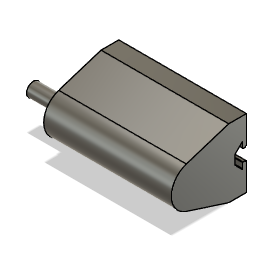
Washer Support v6 (Autodesk Fusion 360 design; units mm, degrees)
Autodesk Fusion 360 part; units mm, degrees
sketch "Sketch1" plane through (0, 0, 0) normal (0, 0, 1) x (1, 0, 0)
  line L0 (0, 0) -> (60, 0)
  line L1 (60, 0) -> (60, 38)
  line L2 (60, 38) -> (0, 38)
  line L3 (0, 38) -> (0, 0)
  point P0 (0, 19)
  dimension "d1" = 38
  dimension "d10" = 60
  constraint horizontal L0
  constraint vertical L1
  constraint horizontal L2
  constraint vertical L3
  constraint coincident L0.start L3.end
  constraint midpoint L3 P0
  measures "d1" distance of L0.start L2.end
  measures "d10" distance of L1.end L2.end
extrude "Extrude1" add sketch "Sketch1" along normal blind 57 makes body 1
sketch "Sketch2" plane through (0, 0, 0) normal (-1, 0, 0) x (0, 0, 1)
  line L0 (0, 38) -> (0, 0)
  line L1 (0, 0) -> (57, 0)
  line L2 (57, 0) -> (57, 38)
  line L3 (57, 38) -> (0, 38)
  line L4 (0, 38) -> (57, 0) construction
  circle A0 centre (28.5, 19) radius 3.85
  line L5 (0, 10) -> (0, 38)
  line L6 (57, 38) -> (0, 38)
  line L7 (57, 38) -> (57, 10)
  line L8 (28.5, 15.15) -> (57, 15.15) construction
  line L9 (28.5, 22.85) -> (57, 22.85) construction
  line L10 (9.8511, 38) -> (57, 22.85)
  line L11 (9.8511, 0) -> (57, 15.15)
  line L12 (57, 22.85) -> (33.4265, 30.4247)
  line L13 (57, 15.15) -> (33.4265, 7.5753)
  arc A1 (33.4265, 7.5753) -> (33.4265, 30.4247) centre (29.7555, 19) ccw
  line L14 (0, 38) -> (57, 38)
  line L15 (57, 38) -> (57, 0)
  line L16 (57, 0) -> (0, 0)
  line L17 (0, 0) -> (0, 38)
  point P0 (9.8511, 38)
  point P1 (9.8511, 0)
  dimension "d4" = 7.7
  dimension "d11" = 12
  constraint coincident L0.start L3.end
  constraint coincident L1.end L2.start
  constraint midpoint L4 A0.centre
  constraint coincident L0 L5.start
  constraint coincident L2 L7.end
  constraint coincident L2.end L3.start
  constraint coincident L6 P0
  constraint coincident L1 P1
  constraint coincident A0 L8.start
  constraint coincident L7 L8.end
  constraint coincident A0 L9.start
  constraint coincident L7 L9.end
  constraint perpendicular L7 L9
  constraint perpendicular L7 L8
  constraint tangent A0 L9
  constraint tangent A0 L8
  constraint coincident P0 L10.start
  constraint coincident P1 L11.start
  constraint collinear L10 L12
  constraint collinear L11 L13
  constraint tangent L13 A1
  constraint tangent L12 A1
  constraint horizontal L14
  constraint vertical L15
  constraint horizontal L16
  constraint vertical L17
  measures "d4" diameter of A0
  measures "d11" radius of A1
extrude "Extrude2" add sketch "Sketch2" along normal blind 19 contours A0 bodies 1
extrude "Extrude4" cut sketch "Sketch2" against normal blind 93 contours L2 L3 L6 L7 L10 L12 L14 L15 | L2 L7 L10 L11 L12 L13 A1 L15 | L1 L2 L7 L11 L13 L15 L16 bodies 1
sketch "profile" plane through (0, 0, 0) normal (0, 1, 0) x (1, 0, 0) in component "20 mm x 20 mm T-Slot v1"
  circle A0 centre (0, 0) radius 2.5
  line L0 (0, -3.9) -> (-2.5, -3.9)
  line L1 (4, -4) -> (-4, 4) construction
  line L2 (-3.9092, -3.9092) -> (4, 4) construction
  line L3 (10, -10) -> (-10, -10) construction
  line L4 (-10, -10) -> (-10, 10) construction
  line L5 (-10, 10) -> (10, 10) construction
  line L6 (10, 10) -> (10, -10) construction
  line L7 (10, -10) -> (-10, 10) construction
  line L8 (-10, -10) -> (10, 10) construction
  line L9 (8, -8) -> (-8, -8) construction
  line L10 (-8, -8) -> (-8, 8) construction
  line L11 (-8, 8) -> (8, 8) construction
  line L12 (8, 8) -> (8, -8) construction
  line L13 (8, -8) -> (-8, 8) construction
  line L14 (-8, -8) -> (8, 8) construction
  line L15 (0, -8) -> (0, -10) construction
  line L16 (0, -9) -> (-3.1, -9) construction
  line L17 (-3.1, -8) -> (-3.1, -9.6)
  line L18 (-1.75, -10) -> (-1.75, -9.6) construction
  line L19 (0, -9.6) -> (-3.5, -9.6) construction
  line L20 (-3.1, -9.6) -> (-3.5, -9.6)
  line L21 (-3.5, -9.6) -> (-3.5, -10)
  line L22 (0, 0) -> (0, -8) construction
  line L23 (-3.5, -10) -> (-10, -10)
  line L24 (-3.9092, -3.9092) -> (-2.5, -3.9) construction
  line L25 (-8, -8) -> (-6.6, -8) construction
  line L26 (-8, -8) -> (-8, -7) construction
  line L27 (-2.5, -3.9) -> (-6.6, -8)
  line L28 (-6.6, -8) -> (-3.1, -8)
  line L29 (0, -2.5) -> (0, -3.9) construction
  line L30 (-3.9, 0) -> (-3.9, -2.5)
  line L31 (-3.9, -2.5) -> (-8, -6.6)
  line L32 (-8, -6.6) -> (-8, -3.1)
  line L33 (-8, -3.1) -> (-9.6, -3.1)
  line L34 (-9.6, -3.1) -> (-9.6, -3.5)
  line L35 (-9.6, -3.5) -> (-10, -3.5)
  line L36 (-10, -3.5) -> (-10, -10)
  line L37 (0, 0) -> (10, 0) construction
  line L38 (3.9, 0) -> (3.9, -2.5)
  line L39 (3.9, -2.5) -> (8, -6.6)
  line L40 (8, -6.6) -> (8, -3.1)
  line L41 (8, -3.1) -> (9.6, -3.1)
  line L42 (9.6, -3.1) -> (9.6, -3.5)
  line L43 (9.6, -3.5) -> (10, -3.5)
  line L44 (10, -3.5) -> (10, -10)
  line L45 (0, -3.9) -> (2.5, -3.9)
  line L46 (6.6, -8) -> (3.1, -8)
  line L47 (3.1, -8) -> (3.1, -9.6)
  line L48 (3.1, -9.6) -> (3.5, -9.6)
  line L49 (3.5, -9.6) -> (3.5, -10)
  line L50 (3.5, -10) -> (10, -10)
  line L51 (2.5, -3.9) -> (6.6, -8)
  line L52 (-3.9, 0) -> (-3.9, 2.5)
  line L53 (-3.9, 2.5) -> (-8, 6.6)
  line L54 (-8, 6.6) -> (-8, 3.1)
  line L55 (-8, 3.1) -> (-9.6, 3.1)
  line L56 (-9.6, 3.1) -> (-9.6, 3.5)
  line L57 (-9.6, 3.5) -> (-10, 3.5)
  line L58 (-10, 3.5) -> (-10, 10)
  line L59 (0, 3.9) -> (-2.5, 3.9)
  line L60 (-6.6, 8) -> (-3.1, 8)
  line L61 (-3.1, 8) -> (-3.1, 9.6)
  line L62 (-3.1, 9.6) -> (-3.5, 9.6)
  line L63 (-3.5, 9.6) -> (-3.5, 10)
  line L64 (-3.5, 10) -> (-10, 10)
  line L65 (-2.5, 3.9) -> (-6.6, 8)
  line L66 (0, 3.9) -> (2.5, 3.9)
  line L67 (6.6, 8) -> (3.1, 8)
  line L68 (3.1, 8) -> (3.1, 9.6)
  line L69 (3.1, 9.6) -> (3.5, 9.6)
  line L70 (3.5, 9.6) -> (3.5, 10)
  line L71 (3.5, 10) -> (10, 10)
  line L72 (2.5, 3.9) -> (6.6, 8)
  line L73 (3.9, 0) -> (3.9, 2.5)
  line L74 (8, 6.6) -> (8, 3.1)
  line L75 (8, 3.1) -> (9.6, 3.1)
  line L76 (9.6, 3.1) -> (9.6, 3.5)
  line L77 (9.6, 3.5) -> (10, 3.5)
  line L78 (10, 3.5) -> (10, 10)
  line L79 (3.9, 2.5) -> (8, 6.6)
  dimension "d3_1" = 5
  dimension "d7" = 8
  dimension "d8" = 8
  dimension "d9" = 20
  dimension "d10_1" = 20
  dimension "d11_1" = 16
  dimension "d12_1" = 16
  dimension "d13_1" = 3.1
  dimension "d14" = 0.4
  dimension "d15" = 3.5
  dimension "d20" = 2.5
  dimension "d21" = 1.4
  constraint coincident A0.centre L22.start
  constraint horizontal L0
  constraint coincident L1 A0.centre
  constraint coincident L2 A0.centre
  constraint horizontal L3
  constraint perpendicular L3 L4
  constraint parallel L3 L5
  constraint parallel L4 L6
  constraint coincident L7 A0.centre
  constraint coincident L8 A0.centre
  constraint horizontal L9
  constraint perpendicular L9 L10
  constraint parallel L9 L11
  constraint parallel L10 L12
  constraint coincident L13 A0.centre
  constraint coincident L14 A0.centre
  constraint midpoint L9 L15.start
  constraint midpoint L3 L15.end
  constraint midpoint L15 L16.start
  constraint perpendicular L15 L16
  constraint coincident L9 L17.start
  constraint perpendicular L3 L17
  constraint coincident L16.end L17
  constraint vertical L18
  constraint coincident L3 L18.start
  constraint coincident L15 L19.start
  constraint perpendicular L15 L19
  constraint coincident L18.end L19
  constraint coincident L19 L17.end
  constraint coincident L3 L21.end
  constraint perpendicular L3 L21
  constraint midpoint L18.end L19
  constraint coincident L9 L25.end
  constraint coincident L10 L26.end
  constraint parallel L14 L27
  constraint coincident L22 L0.start
  constraint coincident L22 L29.start
  constraint coincident A0 L29.start
  constraint parallel L22 L29
  constraint coincident L0.start L29.end
  constraint symmetric L3.end L8 L4.start
  constraint symmetric L8 L17.start L32.end
  constraint symmetric L8 L19.end L34.end
  constraint symmetric L8 L17.end L33.end
  constraint symmetric L8 L21.end L35.end
  constraint symmetric L8 L0.end L30.end
  constraint symmetric L8 L25.end L31.end
  constraint symmetric L8 L0.start L30.start
  constraint midpoint L6 L37.end
  constraint symmetric L3.end L22 L3.start
  constraint symmetric L17.start L22 L46.end
  constraint symmetric L19.end L22 L48.end
  constraint symmetric L17.end L22 L47.end
  constraint symmetric L21.end L22 L49.end
  constraint symmetric L22 L0.end L45.end
  constraint symmetric L22 L25.end L46.start
  constraint symmetric L22 L0.start L29.end
  constraint symmetric L22 L30.start L38.start
  constraint symmetric L22 L30.end L38.end
  constraint symmetric L22 L31.end L39.end
  constraint symmetric L22 L32.end L40.end
  constraint symmetric L22 L33.end L41.end
  constraint symmetric L22 L34.end L42.end
  constraint symmetric L22 L35.end L43.end
  constraint symmetric L22 L3.end L3.start
  constraint symmetric L3.end L37 L4.end
  constraint symmetric L17.start L37 L60.end
  constraint symmetric L19.end L37 L62.end
  constraint symmetric L17.end L37 L61.end
  constraint symmetric L21.end L37 L63.end
  constraint symmetric L0.end L37 L59.end
  constraint symmetric L25.end L37 L60.start
  constraint symmetric L0.start L37 L59.start
  constraint symmetric L30.start L37 L52.start
  constraint symmetric L30.end L37 L52.end
  constraint symmetric L31.end L37 L53.end
  constraint symmetric L32.end L37 L54.end
  constraint symmetric L33.end L37 L55.end
  constraint symmetric L34.end L37 L56.end
  constraint symmetric L35.end L37 L57.end
  constraint symmetric L37 L38.start L73.start
  constraint symmetric L37 L38.end L73.end
  constraint symmetric L37 L39.end L74.start
  constraint symmetric L37 L40.end L74.end
  constraint symmetric L37 L41.end L75.end
  constraint symmetric L37 L42.end L76.end
  constraint symmetric L37 L43.end L77.end
  constraint symmetric L37 L3.start L5.end
  constraint symmetric L37 L0.start L59.start
  constraint symmetric L37 L45.end L66.end
  constraint symmetric L37 L46.start L67.start
  constraint symmetric L37 L46.end L67.end
  constraint symmetric L37 L47.end L68.end
  constraint symmetric L37 L48.end L69.end
  constraint symmetric L37 L49.end L70.end
  measures "d3_1" diameter of A0
  measures "d7" distance of L1.end L2.end
  measures "d8" distance of L1.start L2.end
  measures "d9" distance of L4.end L5.end
  measures "d10_1" distance of L3.end L4.end
  measures "d11_1" distance of L10.end L11.end
  measures "d12_1" distance of L9.end L10.end
  measures "d13_1" distance of L16.start L16.end
  measures "d14" distance of L18.start L18.end
  measures "d15" distance of L19.start L19.end
  measures "d20" distance of L0.end L0.start
  measures "d21" distance of L29.start L0.start
extrude "Extrude3" add sketch "profile" along normal blind 10 separate body makes body 2 in component "20 mm x 20 mm T-Slot v1"
fillet "Fillet1" radius 0.6 4 edges at (-10, 5, 10) (10, 5, 10) (10, 5, -10) (-10, 5, -10) on bodies 2 in component "20 mm x 20 mm T-Slot v1"
fillet "Fillet1" radius 0.2 8 edges at (3.1, 5, 8) (8, 5, 3.1) (8, 5, -3.1) (3.1, 5, -8) (-3.1, 5, 8) (-8, 5, 3.1) (-3.1, 5, -8) (-8, 5, -3.1) on bodies 2 in component "20 mm x 20 mm T-Slot v1"
fillet "Fillet1" radius 0.2 8 edges at (-8, 5, 6.6) (-6.6, 5, 8) (6.6, 5, 8) (8, 5, 6.6) (8, 5, -6.6) (6.6, 5, -8) (-6.6, 5, -8) (-8, 5, -6.6) on bodies 2 in component "20 mm x 20 mm T-Slot v1"
fillet "Fillet1" radius 0.4 8 edges at (-2.5, 5, 3.9) (2.5, 5, 3.9) (3.9, 5, 2.5) (3.9, 5, -2.5) (2.5, 5, -3.9) (-2.5, 5, -3.9) (-3.9, 5, -2.5) (-3.9, 5, 2.5) on bodies 2 in component "20 mm x 20 mm T-Slot v1"
scale "Scale1" factor 1.05 about (-2.3343, 10, 3.9) bodies 2 in component "20 mm x 20 mm T-Slot v1"
sketch "Sketch3" plane through (85, 0, 0) normal (1, 0, 0) x (0, 0, -1)
  arc A0 (-7.21, 27.4933) -> (-7, 27.2833) centre (-7, 27.4933) ccw
  line L0 (-7, 27.2833) -> (-4.042, 27.2833)
  arc A1 (-3.8935, 26.9248) -> (-4.042, 27.2833) centre (-4.042, 27.0733) ccw
  line L1 (-3.8935, 26.9248) -> (-7.717, 23.1013)
  arc A2 (-8.014, 22.9783) -> (-7.717, 23.1013) centre (-8.014, 23.3983) ccw
  line L2 (-8.014, 22.9783) -> (-12.916, 22.9783)
  arc A3 (-13.213, 23.1013) -> (-12.916, 22.9783) centre (-12.916, 23.3983) ccw
  line L3 (-13.213, 23.1013) -> (-17.0365, 26.9248)
  arc A4 (-16.888, 27.2833) -> (-17.0365, 26.9248) centre (-16.888, 27.0733) ccw
  line L4 (-16.888, 27.2833) -> (-13.93, 27.2833)
  arc A5 (-13.93, 27.2833) -> (-13.72, 27.4933) centre (-13.93, 27.4933) ccw
  line L5 (-13.72, 27.4933) -> (-13.72, 28.9633)
  line L6 (-13.72, 28.9633) -> (-14.14, 28.9633)
  line L7 (-14.14, 28.9633) -> (-14.14, 29.3833)
  line L8 (-14.14, 29.3833) -> (-20.335, 29.3833)
  arc A6 (-20.335, 29.3833) -> (-20.965, 28.7533) centre (-20.335, 28.7533) ccw
  line L9 (-20.965, 28.7533) -> (-20.965, 22.5583)
  line L10 (-20.965, 22.5583) -> (-20.545, 22.5583)
  line L11 (-20.545, 22.5583) -> (-20.545, 22.1383)
  line L12 (-20.545, 22.1383) -> (-19.075, 22.1383)
  arc A7 (-19.075, 22.1383) -> (-18.865, 22.3483) centre (-19.075, 22.3483) ccw
  line L13 (-18.865, 22.3483) -> (-18.865, 25.3063)
  arc A8 (-18.5065, 25.4548) -> (-18.865, 25.3063) centre (-18.655, 25.3063) ccw
  line L14 (-18.5065, 25.4548) -> (-14.683, 21.6313)
  arc A9 (-14.56, 21.3343) -> (-14.683, 21.6313) centre (-14.98, 21.3343) ccw
  line L15 (-14.56, 21.3343) -> (-14.56, 16.4323)
  arc A10 (-14.683, 16.1353) -> (-14.56, 16.4323) centre (-14.98, 16.4323) ccw
  line L16 (-14.683, 16.1353) -> (-18.5065, 12.3118)
  arc A11 (-18.865, 12.4603) -> (-18.5065, 12.3118) centre (-18.655, 12.4603) ccw
  line L17 (-18.865, 12.4603) -> (-18.865, 15.4183)
  arc A12 (-18.865, 15.4183) -> (-19.075, 15.6283) centre (-19.075, 15.4183) ccw
  line L18 (-19.075, 15.6283) -> (-20.545, 15.6283)
  line L19 (-20.545, 15.6283) -> (-20.545, 15.2083)
  line L20 (-20.545, 15.2083) -> (-20.965, 15.2083)
  line L21 (-20.965, 15.2083) -> (-20.965, 9.0133)
  arc A13 (-20.965, 9.0133) -> (-20.335, 8.3833) centre (-20.335, 9.0133) ccw
  line L22 (-20.335, 8.3833) -> (-14.14, 8.3833)
  line L23 (-14.14, 8.3833) -> (-14.14, 8.8033)
  line L24 (-14.14, 8.8033) -> (-13.72, 8.8033)
  line L25 (-13.72, 8.8033) -> (-13.72, 10.2733)
  arc A14 (-13.72, 10.2733) -> (-13.93, 10.4833) centre (-13.93, 10.2733) ccw
  line L26 (-13.93, 10.4833) -> (-16.888, 10.4833)
  arc A15 (-17.0365, 10.8418) -> (-16.888, 10.4833) centre (-16.888, 10.6933) ccw
  line L27 (-17.0365, 10.8418) -> (-13.213, 14.6653)
  arc A16 (-12.916, 14.7883) -> (-13.213, 14.6653) centre (-12.916, 14.3683) ccw
  line L28 (-12.916, 14.7883) -> (-8.014, 14.7883)
  arc A17 (-7.717, 14.6653) -> (-8.014, 14.7883) centre (-8.014, 14.3683) ccw
  line L29 (-7.717, 14.6653) -> (-3.8935, 10.8418)
  arc A18 (-4.042, 10.4833) -> (-3.8935, 10.8418) centre (-4.042, 10.6933) ccw
  line L30 (-4.042, 10.4833) -> (-7, 10.4833)
  arc A19 (-7, 10.4833) -> (-7.21, 10.2733) centre (-7, 10.2733) ccw
  line L31 (-7.21, 10.2733) -> (-7.21, 8.8033)
  line L32 (-7.21, 8.8033) -> (-6.79, 8.8033)
  line L33 (-6.79, 8.8033) -> (-6.79, 8.3833)
  line L34 (-6.79, 8.3833) -> (-0.595, 8.3833)
  arc A20 (-0.595, 8.3833) -> (0.035, 9.0133) centre (-0.595, 9.0133) ccw
  line L35 (0.035, 9.0133) -> (0.035, 15.2083)
  line L36 (0.035, 15.2083) -> (-0.385, 15.2083)
  line L37 (-0.385, 15.2083) -> (-0.385, 15.6283)
  line L38 (-0.385, 15.6283) -> (-1.855, 15.6283)
  arc A21 (-1.855, 15.6283) -> (-2.065, 15.4183) centre (-1.855, 15.4183) ccw
  line L39 (-2.065, 15.4183) -> (-2.065, 12.4603)
  arc A22 (-2.4235, 12.3118) -> (-2.065, 12.4603) centre (-2.275, 12.4603) ccw
  line L40 (-2.4235, 12.3118) -> (-6.247, 16.1353)
  arc A23 (-6.37, 16.4323) -> (-6.247, 16.1353) centre (-5.95, 16.4323) ccw
  line L41 (-6.37, 16.4323) -> (-6.37, 21.3343)
  arc A24 (-6.247, 21.6313) -> (-6.37, 21.3343) centre (-5.95, 21.3343) ccw
  line L42 (-6.247, 21.6313) -> (-2.4235, 25.4548)
  arc A25 (-2.065, 25.3063) -> (-2.4235, 25.4548) centre (-2.275, 25.3063) ccw
  line L43 (-2.065, 25.3063) -> (-2.065, 22.3483)
  arc A26 (-2.065, 22.3483) -> (-1.855, 22.1383) centre (-1.855, 22.3483) ccw
  line L44 (-1.855, 22.1383) -> (-0.385, 22.1383)
  line L45 (-0.385, 22.1383) -> (-0.385, 22.5583)
  line L46 (-0.385, 22.5583) -> (0.035, 22.5583)
  line L47 (0.035, 22.5583) -> (0.035, 28.7533)
  arc A27 (0.035, 28.7533) -> (-0.595, 29.3833) centre (-0.595, 28.7533) ccw
  line L48 (-0.595, 29.3833) -> (-6.79, 29.3833)
  line L49 (-6.79, 29.3833) -> (-6.79, 28.9633)
  line L50 (-6.79, 28.9633) -> (-7.21, 28.9633)
  line L51 (-7.21, 28.9633) -> (-7.21, 27.4933)
  circle A28 centre (-10.465, 18.8833) radius 2.625
  line L52 (0.035, 22.5583) -> (0.035, 15.2083)
  constraint coincident L46.end L47.start
  constraint coincident L35.end L36.start
extrude "Extrude5" cut sketch "Sketch3" against normal blind 100 contours L36 L37 L38 A21 L39 A22 L40 A23 L41 A24 L42 A25 L43 A26 L44 L45 L46 L52 bodies 1
extrude "Extrude6" add 1 faces at (60, 19.7781, 24.4077) along direction (1, 0, 0) blind 11 on bodies 1 bodies 1
sketch "Sketch4" plane through (0, 0, 0) normal (-1, 0, 0) x (0, 0, 1)
  line L0 (0.385, 15.2083) -> (0, 15.2083)
  line L1 (0, 15.2083) -> (0, 0)
  line L2 (0, 0) -> (9.8511, 0)
  line L3 (9.8511, 0) -> (33.4265, 7.5753)
  arc A0 (33.4265, 7.5753) -> (33.4265, 30.4247) centre (29.7555, 19) ccw
  line L4 (33.4265, 30.4247) -> (9.8511, 38)
  line L5 (9.8511, 38) -> (0, 38)
  line L6 (0, 38) -> (0, 22.5583)
  line L7 (0, 22.5583) -> (0.385, 22.5583)
  line L8 (0.385, 22.5583) -> (0.385, 22.1383)
  line L9 (0.385, 22.1383) -> (1.855, 22.1383)
  arc A1 (1.855, 22.1383) -> (2.065, 22.3483) centre (1.855, 22.3483) ccw
  line L10 (2.065, 22.3483) -> (2.065, 25.3063)
  arc A2 (2.4235, 25.4548) -> (2.065, 25.3063) centre (2.275, 25.3063) ccw
  line L11 (2.4235, 25.4548) -> (6.247, 21.6313)
  arc A3 (6.37, 21.3343) -> (6.247, 21.6313) centre (5.95, 21.3343) ccw
  line L12 (6.37, 21.3343) -> (6.37, 16.4323)
  arc A4 (6.247, 16.1353) -> (6.37, 16.4323) centre (5.95, 16.4323) ccw
  line L13 (6.247, 16.1353) -> (2.4235, 12.3118)
  arc A5 (2.065, 12.4603) -> (2.4235, 12.3118) centre (2.275, 12.4603) ccw
  line L14 (2.065, 12.4603) -> (2.065, 15.4183)
  arc A6 (2.065, 15.4183) -> (1.855, 15.6283) centre (1.855, 15.4183) ccw
  line L15 (1.855, 15.6283) -> (0.385, 15.6283)
  line L16 (0.385, 15.6283) -> (0.385, 15.2083)
  circle A7 centre (28.5, 19) radius 3.85
  circle A8 centre (28.5, 19) radius 5.85
  dimension "d23" = 2
extrude "Extrude7" add sketch "Sketch4" along normal blind 0.5 contours A8 bodies 1
chamfer "Chamfer1" distance 0.1 angle 45 1 edges at (-0.5, 16.8845, 23.0459) on bodies 1
component "20 mm x 20 mm T-Slot v1" placed x (0, -1, 0) y (1, 0, 0) z (0, 0, 1) at (75, 19, 10.66)
equation "d13_1 = ( 6.2 / 2 ) * 1 mm"
equation "d15 = 7 mm / 2"
